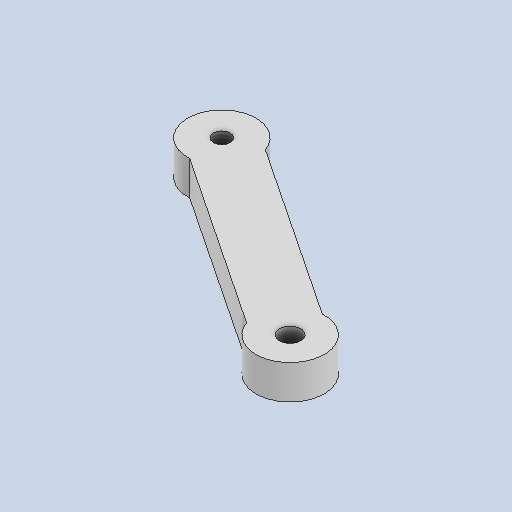
# Autodesk Inventor part: gripper_hand_connector
Saved by Autodesk Inventor 2024 (Build 280153000, 153)
## iProperties
Created: 2023-09-08
Part Number: gripper_hand_connector
Material: Generic
Document SubType Name: Modeling
Designer: 박동준
Density: 1 g/cm^3
Appearance: Default
Author: 박동준
Autodesk Inventor part; units mm, degrees
ref_plane "YZ Plane" through (0, 0, 0) normal (1, 0, 0) x (0, 1, 0)
ref_plane "XZ Plane" through (0, 0, 0) normal (0, 1, 0) x (-1, 0, 0)
ref_plane "XY Plane" through (0, 0, 0) normal (0, 0, 1) x (1, 0, 0)
sketch "Sketch1" plane through (0, 0, 0) normal (0, 1, 0) x (-1, 0, 0)
  circle A0 centre (0, 0) radius 5
  circle A1 centre (-30, 20) radius 5
  line L0 (-4.715, -1.6641) -> (-29.7226, 15.0077)
  line L1 (-0.2774, 4.9923) -> (-25.285, 21.6641)
  line L2 (0, 0) -> (-30, 0) construction
  line L3 (-30, 0) -> (-30, 20) construction
  line L4 (0, 0) -> (-30, 20) construction
  dimension "d0" = 10
  dimension "d1" = 10
  dimension "d2" = 4
  dimension "d3" = 4
  dimension "d4" = 30
  dimension "d5" = 20
  constraints: 10 end point, 4 point on circle, 2 centre point, 2 parallel, 1 coincident, 1 horizontal, 1 perpendicular
  measures "d0" diameter of A0
  measures "d1" diameter of A1
  measures "d2" distance between parallel lines of L0 L4
  measures "d3" distance between parallel lines of L1 L4
  measures "d4" distance of L2.start L2.end
  measures "d5" distance of L2.end L3.end
extrude "Extrusion1" add sketch "Sketch1" along normal blind 5
sketch "Sketch2" plane through (0, 0, 0) normal (0, -1, 0) x (1, 0, 0)
  line L0 (0, 0) -> (30, 20) construction
  arc A0 (29.7226, 15.0077) -> (25.285, 21.6641) centre (30, 20) ccw projected
  line L1 (0.2774, 4.9923) -> (25.285, 21.6641) projected
  arc A1 (0.2774, 4.9923) -> (4.715, -1.6641) centre (0, 0) ccw projected
  line L2 (29.7226, 15.0077) -> (4.715, -1.6641) projected
  constraints: 2 coincident
hole "Hole1" at (30, 0, 20) direction (0, 1, 0) diameter 3.1 end through all
ref_plane "Work Plane1" through (0, 1.5, 0) normal (0, 1, 0) x (1, 0, 0)
sketch "Sketch4" plane through (0, 5, 0) normal (0, 1, 0) x (1, 0, 0)
  circle A0 centre (30, -20) radius 1.55 projected
  arc A1 (25.285, -21.6641) -> (29.7226, -15.0077) centre (30, -20) ccw projected
  line L0 (29.7226, -15.0077) -> (4.715, 1.6641) projected
  arc A2 (4.715, 1.6641) -> (0.2774, -4.9923) centre (0, 0) ccw projected
  line L1 (0.2774, -4.9923) -> (25.285, -21.6641) projected
  constraints: 1 coincident
hole "Hole2" at (0, 5, 0) direction (0, -1, 0) diameter 2.459 end through all thread size "M3x0.5" class "6H" standard "ISO Metric profile"
body "Solid1"
